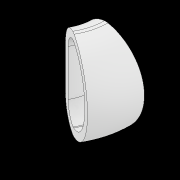
# Autodesk Inventor part: L_Filt1-Wedge
Saved by Autodesk Inventor 2021 (Build 250183000, 183)
## iProperties
Created: 2020-11-13
Part Number: L_Filt1-Wedge
Material: UHMW, White
Document SubType Name: Modeling
Designer: Eli Mattingly
Density: 0.94 g/cm^3
Appearance: Smooth - White
Author: Eli Mattingly
Autodesk Inventor part; units mm, degrees
ref_plane "Work Plane1" through (-7, 0, -29.5697) normal (1, 0, 0) x (0, 0, -1)
ref_plane "YZ Plane" through (0, 0, 0) normal (1, 0, 0) x (0, 1, 0)
ref_plane "XZ Plane" through (0, 0, 0) normal (0, 1, 0) x (-1, 0, 0)
sketch "Sketch1" plane through (0, 0, 0) normal (0, 0, 1) x (1, 0, 0)
  line L0 (0, 0) -> (0, 18.76) construction
  line L1 (12.505, 9.605) -> (12.505, -9.605)
  line L2 (21.66, 18.76) -> (21.66, -18.76) construction
  arc A0 (20.8454, 18.7237) -> (12.505, 9.605) centre (21.66, 9.605) ccw
  arc A1 (12.505, -9.605) -> (20.8454, -18.7237) centre (21.66, -9.605) ccw
  arc A2 (22.2889, -18.6428) -> (22.2889, 18.6428) centre (18.4889, 0) ccw
  line L3 (0, 0) -> (51.4073, 0)
  arc A3 (22.2889, 18.6428) -> (20.8454, 18.7237) centre (21.2903, 13.7435) ccw
  arc A4 (20.8454, -18.7237) -> (22.2889, -18.6428) centre (21.2903, -13.7435) ccw
  arc A5 (21.6898, 15.7032) -> (21.1123, 15.7356) centre (21.2903, 13.7435) ccw
  arc A6 (21.1123, 15.7356) -> (15.505, 9.605) centre (21.66, 9.605) ccw
  line L4 (15.505, 9.605) -> (15.505, -9.605)
  arc A7 (15.505, -9.605) -> (21.1123, -15.7356) centre (21.66, -9.605) ccw
  arc A8 (21.1123, -15.7356) -> (21.6898, -15.7032) centre (21.2903, -13.7435) ccw
  arc A9 (21.6898, -15.7032) -> (21.6898, 15.7032) centre (18.4889, 0) ccw
  point P0 (12.505, 0)
  point P1 (37.515, 0)
  point P2 (21.66, 0)
  dimension "MaxHeight" = 18.76
  dimension "FlatHeightx2" = 19.21
  dimension "ID" = 25.01
  dimension "OD" = 75.03
  dimension "d5" = 37.52
  dimension "RadAtPeak" = 21.66
  dimension "d90" = 5
  dimension "d97" = 3
  constraints: 25 point on circle, 10 centre point, 10 end point, 5 tangent, 3 horizontal alignment, 3 vertical, 2 line through centre, 2 midpoint, 1 equal radius, 1 horizontal, 5 other
  measures "MaxHeight" distance of L0.start L0.end
  measures "FlatHeightx2" distance of L1.start L1.end
  measures "ID" diameter of L1 L0
  measures "OD" diameter of point (37.515, 0) L0
  measures "d5" distance of L2.start L2.end
  measures "RadAtPeak" distance from line of L0.start L2
  measures "d90" radius of A3
  measures "d97" radial gap between concentric circles of A2 A9
revolve "Revolution1" add sketch "Sketch1" angle 30 about axis through (0, 0, 0) along (0, -1, 0) contours A0 A3 A2 L3 A9 A5 A6 L4 L1 | L3 L4 A7 A8 A9 A2 A4 A1 L1
sketch "Sketch13" plane through (12.505, -9.605, 0) normal (0, 0, -1) x (-1, 0, 0)
  arc A0 (0, 19.21) -> (-8.3404, 28.3287) centre (-9.155, 19.21) ccw projected
  arc A1 (-8.3404, 28.3287) -> (-9.7839, 28.2478) centre (-8.7853, 23.3485) ccw projected
  arc A2 (-9.7839, 28.2478) -> (-9.8497, 28.2342) centre (-5.9839, 9.605) ccw projected
  arc A3 (-9.7839, -9.0378) -> (-8.3404, -9.1187) centre (-8.7853, -4.1385) ccw projected
  arc A4 (-8.3404, -9.1187) -> (0, 0) centre (-9.155, 0) ccw projected
  line L0 (0, 19.21) -> (0, 0) projected
  line L1 (-9.155, 0) -> (3, 0)
  line L2 (3, 0) -> (3, 19.21)
  line L3 (3, 19.21) -> (-9.155, 19.21)
  line L4 (-9.155, 19.21) -> (-9.155, 0)
  arc A5 (-9.8497, 28.2342) -> (-9.8497, -9.0242) centre (-5.9839, 9.605) ccw projected
  point P0 (12.505, 9.605)
  point P1 (-6.673, 9.4777)
  dimension "d93" = 3
  constraints: 8 end point, 2 parallel, 1 horizontal, 1 horizontal alignment, 1 perpendicular, 3 other
  measures "d93" distance between parallel lines of L0 L2
sketch "Sketch7" plane through (0, 0, 0) normal (0, 1, 0) x (-1, 0, 0)
  circle A0 centre (0, 0) radius 198.9616
  constraints: 1 centre point, 1 coincident
sketch "Sketch8" plane through (0, 0, 0) normal (1, 0, 0) x (0, 1, 0)
  circle A0 centre (0, 0) radius 159.0195
  constraints: 1 centre point, 1 coincident
sketch "Sketch9" plane through (0, 0, 0) normal (1, 0, 0) x (0, 0, -1)
  line L0 (74, 0) -> (35, 0) projected
  point P0 (0, 0)
  point P1 (-52.5, 0)
  point P2 (0, 0)
  point P3 (52.5, 0)
  dimension "d88" = 105
  dimension "d89" = 52.5
  constraints: 1 point on line
  measures "d88" distance of point (52.5, 0) point (-52.5, 0)
  measures "d89" distance of point (52.5, 0) point (0, 0)
sketch "Sketch11" plane through (0, 0, 0) normal (1, 0, 0) x (0, 0, -1)
  arc A0 (-35, 25.9107) -> (-42.6927, 34.8921) centre (-44.0893, 25.9107) ccw projected
  line L0 (-35, 25.9107) -> (-35, 0) projected
  line L1 (-35, 0) -> (35, 0) projected
  arc A1 (-50.0415, 0) -> (-54.9585, 0) centre (-52.5, 0) ccw projected
  arc A2 (-50.0415, 0) -> (-54.9585, 0) centre (-37.5, 0) ccw projected
  arc A3 (-39.8678, 39.0634) -> (-73, 0) centre (-33.4058, 0) ccw
  arc A4 (-29.5697, 27.789) -> (-36.4391, 38.3935) centre (-44.0893, 25.9107) ccw
  line L2 (-29.5697, 27.789) -> (-29.5697, 0)
  line L3 (-35, 0) -> (35, 0) projected
  line L4 (-73, 0) -> (-29.5697, 0)
  arc A5 (-36.4391, 38.3935) -> (-39.8678, 39.0634) centre (-39.0518, 34.1304) ccw
  point P0 (0, 0)
  point P1 (-35, 0)
  point P2 (-29.5697, 0)
  point P3 (-54.9585, 0)
  point P4 (-50.0415, 0)
  dimension "d91" = 5
  constraints: 6 point on circle, 4 end point, 3 centre point, 2 tangent, 1 horizontal, 1 point on line, 1 other
  measures "d91" radius of A5
sketch "Sketch6" plane through (2.8986, 0, 1.6735) normal (-0.5, 0, 0.866) x (0, 1, 0)
  line L0 (-9.605, -9.1579) -> (9.605, -9.1579) projected
  arc A0 (-18.6428, -18.9419) -> (18.6428, -18.9419) centre (0, -15.1418) ccw projected
  arc A1 (-20.0253, -21.5516) -> (20.0253, -21.5516) centre (0, -15.1418) ccw
  line L1 (18.6428, -18.9419) -> (18.1205, -18.9419)
  arc A2 (20.0253, -21.5516) -> (18.1205, -18.9419) centre (18.1205, -20.9419) ccw
  line L2 (-18.1205, -18.9419) -> (-18.6428, -18.9419)
  arc A3 (-18.1205, -18.9419) -> (-20.0253, -21.5516) centre (-18.1205, -20.9419) ccw
  line L3 (-28.9637, 3.3471) -> (28.9637, 3.3471) projected
  point P0 (0, 3.3471)
  point P1 (-20.6799, -18.9419)
  point P2 (20.6799, -18.9419)
  point P3 (18.6292, -19.0077)
  point P4 (-18.6292, -19.0077)
  dimension "d47" = 2
  dimension "d48" = 2
  dimension "d49" = 2
  constraints: 8 point on circle, 4 end point, 4 tangent, 3 centre point, 2 point on line, 1 horizontal
  measures "d47" radial gap between concentric circles of A0 A1
  measures "d48" radius of A2
  measures "d49" radius of A3
equation "\"d5\" = 2 * MaxHeight"
equation "\"d63_Copy\" = 35"
body "Solid1"
